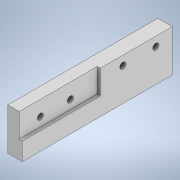
# Autodesk Inventor part: bodybottompart
Saved by Autodesk Inventor 2020.3 (Build 243373000, 373)
## iProperties
Created: 2021-06-21
Part Number: bodybottompart
Material: Generic
Document SubType Name: Modeling
Designer: 0x6f736f646f
Density: 1 g/cm^3
Appearance: Default
Author: 0x6f736f646f
Autodesk Inventor part; units mm, degrees
ref_plane "YZ Plane" through (0, 0, 0) normal (1, 0, 0) x (0, 1, 0)
ref_plane "XZ Plane" through (0, 0, 0) normal (0, 1, 0) x (-1, 0, 0)
ref_plane "XY Plane" through (0, 0, 0) normal (0, 0, 1) x (1, 0, 0)
sketch "Sketch1" plane through (0, 0, 0) normal (1, 0, 0) x (0, 1, 0)
  line L0 (0, 0) -> (70, 0)
  line L1 (70, 0) -> (70, 250)
  line L2 (70, 250) -> (0, 250)
  line L3 (0, 250) -> (0, 0)
  line L4 (70, 250) -> (30, 250)
  line L5 (30, 250) -> (30, 120)
  line L6 (30, 120) -> (70, 120)
  line L7 (70, 120) -> (70, 250)
  circle A0 centre (45, 215) radius 5
  circle A1 centre (45, 165) radius 5
  circle A2 centre (55, 82.5) radius 5
  circle A3 centre (55, 27.5) radius 5
  dimension "d0" = 70
  dimension "d1" = 250
  dimension "d2" = 50
  dimension "d3" = 10
  dimension "d4" = 25
  dimension "d5" = 130
  dimension "d6" = 40
  dimension "d7" = 35
  dimension "d12" = 10
  dimension "d13" = 15
  dimension "d14" = 55
  dimension "d15" = 27.5
  constraints: 16 end point, 4 centre point, 4 parallel, 2 equal radius, 2 horizontal, 2 perpendicular, 2 vertical alignment
  measures "d0" distance of L2.end L1.end
  measures "d1" distance of L1.end L0.end
  measures "d2" distance of A1.centre A0.centre
  measures "d3" diameter of A0
  measures "d4" distance from line of A0.centre L1
  measures "d5" distance of L4.end L5.end
  measures "d6" distance between parallel lines of L5 L1
  measures "d7" distance from line of L2 A0.centre
  measures "d12" diameter of A3
  measures "d13" distance from line of A3.centre L1
  measures "d14" distance of A2.centre A3.centre
  measures "d15" distance from line of L0 A3.centre
extrude "Extrusion1" add sketch "Sketch1" against normal blind 24.125 contours L3 L2 L5 L6 L1 L0 | L6 L5 L2 L1 | A2 | A3
extrude "Extrusion2" cut sketch "Sketch1" against normal blind 5 contours L6 L5 L2 L1
extrude "Extrusion3" cut sketch "Sketch1" against normal through all contours A2 | A3
body "Solid1"
